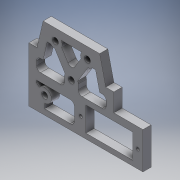
# Autodesk Inventor part: sheet_a
Saved by Autodesk Inventor 2016 (Build 200138000, 138)
## iProperties
Created: 2016-01-11
Part Number: sheet_a
Material: ABS Plastic
Document SubType Name: Modeling
Designer: Nanjar
Density: 1.06 g/cm^3
Appearance: Smooth - White
Author: Nanjar
Autodesk Inventor part; units mm, degrees
ref_plane "YZ Plane" through (0, 0, 0) normal (1, 0, 0) x (0, 1, 0)
ref_plane "XZ Plane" through (0, 0, 0) normal (0, 1, 0) x (-1, 0, 0)
ref_plane "XY Plane" through (0, 0, 0) normal (0, 0, 1) x (1, 0, 0)
sketch "Sketch1" plane through (0, 0, 0) normal (0, 0, 1) x (1, 0, 0)
  line L0 (11.5, -6) -> (-11.5, -6)
  line L1 (-11.5, -6) -> (-11.5, 6)
  line L2 (-11.5, 6) -> (11.5, 6)
  line L3 (11.5, 6) -> (11.5, -6)
  line L4 (16.5, 9.5) -> (16.5, -9.5)
  circle A0 centre (-14, 0) radius 0.8
  circle A1 centre (14, 0) radius 0.8
  line L5 (-32.5, 31.2) -> (-4.7599, 31.2)
  line L6 (16.5001, 31.2) -> (16.5, 31.2)
  line L7 (-35.5, 18.42) -> (-39.5, 18.42)
  line L8 (-39.5, 18.42) -> (-35.5, 18.42)
  line L9 (-35.5, 18.42) -> (-32.5, 31.2)
  line L10 (2.2401, 18.42) -> (-1.7599, 18.42)
  line L11 (-1.7599, 18.42) -> (-4.7599, 31.2)
  line L12 (-39.5, 18.42) -> (-39.5, -9.5)
  line L13 (2.2401, 9.5) -> (16.5, 9.5)
  line L14 (16.5, -9.5) -> (-39.5, -9.5)
  line L15 (2.2401, 18.42) -> (2.2401, 9.5)
  point P0 (0, 0)
  point P1 (0, 0)
  dimension "d4" = 1.6
  dimension "d5" = 1.6
  constraints: 32 end point, 2 centre point, 2 horizontal, 2 parallel, 2 perpendicular, 1 point on line, 1 vertical
  measures "d4" diameter of A0
  measures "d5" diameter of A1
extrude "Extrusion1" add sketch "Sketch1" along normal blind 4
sketch "Sketch3" plane through (0, 0, 4) normal (0, 0, 1) x (1, 0, 0)
  circle A0 centre (-26.5, 25.7) radius 1.5
  point P0 (0, 0)
  dimension "d21" = 3
  constraints: 1 centre point
  measures "d21" diameter of A0
extrude "Extrusion3" cut sketch "Sketch3" against normal through all
sketch "Sketch4" plane through (0, 0, 4) normal (0, 0, 1) x (1, 0, 0)
  circle A0 centre (-10.7599, 25.7) radius 1.5
  dimension "d29" = 3
  constraints: 1 centre point
  measures "d29" diameter of A0
extrude "Extrusion4" cut sketch "Sketch4" against normal through all
sketch "Sketch6" plane through (0, 0, 4) normal (0, 0, 1) x (1, 0, 0)
  circle A0 centre (-31.76, 0) radius 1.5
  line L0 (-39.5, -9.5) -> (16.5, -9.5) projected
  line L1 (-39.5, 18.42) -> (-39.5, -9.5) projected
  point P0 (0, 0)
  dimension "d49" = 3
  dimension "d50" = 9.5
  dimension "d51" = 7.74
  constraints: 1 centre point
  measures "d49" diameter of A0
  measures "d50" distance from line of L0 A0.centre
  measures "d51" distance from line of L1 A0.centre
extrude "Extrusion6" cut sketch "Sketch6" against normal through all
sketch "Sketch7" plane through (0, 0, 4) normal (0, 0, 1) x (1, 0, 0)
  circle A0 centre (-18.63, 12.99) radius 1.5
  line L0 (-4.7599, 31.2) -> (-32.5, 31.2) projected
  line L1 (-39.5, 18.42) -> (-39.5, -9.5) projected
  point P0 (0, 0)
  dimension "d54" = 3
  dimension "d55" = 18.21
  dimension "d56" = 20.87
  constraints: 1 centre point
  measures "d54" diameter of A0
  measures "d55" distance from line of L0 A0.centre
  measures "d56" distance from line of L1 A0.centre
extrude "Extrusion7" cut sketch "Sketch7" against normal through all
sketch "Sketch8" plane through (0, 0, 4) normal (0, 0, 1) x (1, 0, 0)
  arc A0 (-31.76, -3.35) -> (-34.3261, 2.1535) centre (-31.76, 0) ccw
  line L0 (-32.5298, 14.6719) -> (-30.4978, 23.3283)
  line L1 (-6.7621, 23.3283) -> (-4.7301, 14.6719)
  line L2 (-4.7301, 14.6719) -> (-1.508, 14.6719)
  line L3 (-1.508, 14.6719) -> (-1.508, 8.6123)
  line L4 (-17.13, -5.7519) -> (-31.76, -5.7519)
  line L5 (-35.7519, 14.6719) -> (-32.5298, 14.6719)
  line L6 (-23.6446, 27.4519) -> (-13.6153, 27.4519)
  line L7 (-15.28, 8.6123) -> (-1.508, 8.6123)
  line L8 (-21.98, 13.105) -> (-21.98, 8.6123)
  line L9 (-21.98, 8.6123) -> (-35.7519, 8.6123)
  line L10 (-17.13, -3.35) -> (-17.13, 4.46)
  line L11 (-17.13, 4.46) -> (-35.7519, 4.46)
  line L12 (-17.13, -3.35) -> (-17.13, -5.7519)
  line L13 (-31.76, -3.35) -> (-31.76, -5.7519)
  line L14 (-35.7519, 3.35) -> (-35.7519, 4.46)
  line L15 (-35.7519, 8.6123) -> (-35.7519, 14.6719)
  line L16 (-35.7519, 3.35) -> (-34.3261, 2.1535)
  line L17 (-28.8659, 23.3283) -> (-30.4978, 23.3283)
  line L18 (-6.7621, 23.3283) -> (-8.394, 23.3283)
  line L19 (-15.28, 13.105) -> (-15.28, 8.6123)
  line L20 (-23.3848, 24.468) -> (-18.63, 16.789)
  line L21 (-18.63, 16.789) -> (-13.8751, 24.468)
  line L22 (-15.5148, 14.222) -> (-10.4743, 22.3622)
  line L23 (-26.7856, 22.3622) -> (-21.7452, 14.222)
  arc A1 (-15.28, 12.99) -> (-15.5148, 14.222) centre (-18.63, 12.99) ccw
  arc A2 (-21.7452, 14.222) -> (-21.98, 12.99) centre (-18.63, 12.99) ccw
  arc A3 (-13.6153, 27.4519) -> (-13.8751, 24.468) centre (-10.7599, 25.7) ccw
  arc A4 (-10.4743, 22.3622) -> (-8.394, 23.3283) centre (-10.7599, 25.7) ccw
  arc A5 (-28.8659, 23.3283) -> (-26.7856, 22.3622) centre (-26.5, 25.7) ccw
  arc A6 (-23.3848, 24.468) -> (-23.6446, 27.4519) centre (-26.5, 25.7) ccw
  dimension "d61" = 6.7
  constraints: 48 end point, 14 point on circle, 7 centre point, 6 point on line, 4 perpendicular, 2 coincident, 2 tangent, 1 horizontal
  measures "d61" diameter of A0
extrude "Extrusion8" cut sketch "Sketch8" against normal blind 10
fillet "Fillet1" radius 2 5 edges at (-35.7519, 8.6123, 2) (-15.28, 8.6123, 2) (-21.98, 8.6123, 2) (-1.508, 8.6123, 2) (-18.63, 16.789, 2)
fillet "Fillet2" radius 2 2 edges at (-1.508, 14.6719, 2) (-35.7519, 14.6719, 2)
fillet "Fillet3" radius 2 2 edges at (-17.13, 4.46, 2) (-17.13, -5.7519, 2)
move faces "Move2" translate (0, 1, 0) faces at (-20.8333, -9.5, 1.3333)
body "Solid1"
